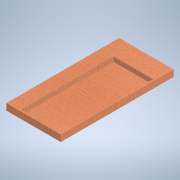
# Autodesk Inventor part: Case stock 1
Saved by Autodesk Inventor 2022 (Build 260153000, 153)
## iProperties
Created: 2022-03-03
Part Number: Case stock 1
Material: Generic
Document SubType Name: Modeling
Designer: Nathan Griffith
Density: 1 g/cm^3
Appearance: White Oak - Natural Medium Gloss
Author: Nathan Griffith
Autodesk Inventor part; units mm, degrees
ref_plane "YZ Plane" through (0, 0, 0) normal (1, 0, 0) x (0, 1, 0)
ref_plane "XZ Plane" through (0, 0, 0) normal (0, 1, 0) x (-1, 0, 0)
ref_plane "XY Plane" through (0, 0, 0) normal (0, 0, 1) x (1, 0, 0)
sketch "Sketch1" plane through (0, 0, 0) normal (0, 1, 0) x (-1, 0, 0)
  line L0 (0, 0) -> (184.15, 0)
  line L1 (184.15, 0) -> (184.15, 381)
  line L2 (184.15, 381) -> (0, 381)
  line L3 (0, 381) -> (0, 0)
  dimension "d0" = 184.15
  dimension "d1" = 381
  constraints: 8 end point, 2 parallel, 1 horizontal, 1 perpendicular
  measures "d0" distance of L2.end L1.end
  measures "d1" distance of L1.end L0.end
extrude "Extrusion1" add sketch "Sketch1" along normal blind 21.6408
sketch "Sketch2" plane through (0, 21.6408, 0) normal (0, 1, 0) x (1, 0, 0)
  line L0 (0, -381) -> (-133.35, -381)
  line L1 (-133.35, -381) -> (-133.35, -57.15)
  line L2 (-133.35, -57.15) -> (0, -57.15)
  line L3 (0, -57.15) -> (0, -381)
  line L4 (0, -381) -> (0, 0) projected
  line L5 (-184.15, -381) -> (0, -381) projected
  dimension "d4" = 133.35
  dimension "d5" = 323.85
  dimension "d6" = 0
  dimension "d7" = 0
  constraints: 8 end point, 2 parallel, 1 horizontal, 1 perpendicular
  measures "d4" distance of L1.end L2.end
  measures "d5" distance of L0.end L1.end
  measures "d6" distance between parallel lines of L4 L3
  measures "d7" distance between parallel lines of L5 L0
extrude "Extrusion2" cut sketch "Sketch2" against normal blind 18.0086
body "Solid1"
